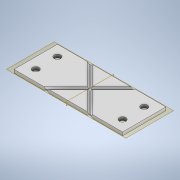
# Autodesk Inventor part: test_hangle_org_1
Saved by Autodesk Inventor 2020 (Build 240168000, 168)
## iProperties
Created: 2021-04-08
Part Number: test_hangle_org_1
Material: Generic
Document SubType Name: Modeling
Designer: Shuang Peng
Density: 1 g/cm^3
Appearance: Default
Author: Shuang Peng
Autodesk Inventor part; units mm, degrees
ref_plane "YZ Plane" through (0, 0, 0) normal (1, 0, 0) x (0, 1, 0)
ref_plane "XZ Plane" through (0, 0, 0) normal (0, 1, 0) x (-1, 0, 0)
ref_plane "XY Plane" through (0, 0, 0) normal (0, 0, 1) x (1, 0, 0)
sketch "Sketch1" plane through (0, 0, 0) normal (0, 1, 0) x (-1, 0, 0)
  line L0 (0, 0) -> (50, 0)
  line L1 (50, 0) -> (50, -20)
  line L2 (50, -20) -> (0, -20)
  line L3 (0, -20) -> (0, 0)
  line L4 (25, 0) -> (25, -20)
  line L5 (25, -20) -> (35, -20)
  line L6 (25, 0) -> (35, 0)
  line L7 (25, 0) -> (15, 0)
  line L8 (25, -20) -> (15, -20)
  line L9 (15, -20) -> (25, -10)
  line L10 (15, 0) -> (25, -10)
  line L11 (25, -10) -> (35, -20)
  line L12 (25, -10) -> (35, 0)
  line L13 (39.318912, 3.965359) -> (38.965359, 4.318912)
  line L14 (38.965359, 4.318912) -> (10.681088, -23.965359)
  line L15 (10.681088, -23.965359) -> (11.034641, -24.318912)
  line L16 (11.034641, -24.318912) -> (39.318912, 3.965359)
  line L17 (39.318912, 3.965359) -> (10.681088, -23.965359) construction
  line L18 (38.965359, 4.318912) -> (11.034641, -24.318912) construction
  line L19 (39.318912, -23.965359) -> (38.965359, -24.318912)
  line L20 (38.965359, -24.318912) -> (10.681088, 3.965359)
  line L21 (10.681088, 3.965359) -> (11.034641, 4.318912)
  line L22 (11.034641, 4.318912) -> (39.318912, -23.965359)
  line L23 (39.318912, -23.965359) -> (10.681088, 3.965359) construction
  line L24 (38.965359, -24.318912) -> (11.034641, 4.318912) construction
  point P0 (14.646447, -20)
  point P1 (24.646447, -10)
  point P2 (14.646447, 0)
  point P3 (35.353553, 0)
  point P4 (25.353553, -10)
  point P5 (35.353553, -20)
  point P6 (25, -10.353553)
  point P7 (15.353553, -20)
  point P8 (34.646447, -20)
  point P9 (15.353553, 0)
  point P10 (25, -9.646447)
  point P11 (34.646447, 0)
  dimension "d0" = 50
  dimension "d1" = 20
  dimension "d2" = 10
  dimension "d3" = 10
  dimension "d4" = 10
  dimension "d5" = 10
  dimension "d6" = 0.5
  dimension "d7" = 40
  dimension "d8" = 0.5
  dimension "d9" = 40
  constraints: 50 end point, 7 midpoint, 6 parallel, 5 perpendicular, 4 point on line, 1 horizontal
  measures "d0" distance of L1.end L2.end
  measures "d1" distance of L0.end L1.end
  measures "d2" distance of L4.end L5.end
  measures "d3" distance of L4.start L6.end
  measures "d4" distance of L4.start L7.end
  measures "d5" distance of L4.end L8.end
  measures "d6" distance of L13.start L13.end
  measures "d7" distance of L14.end L13.end
  measures "d8" distance of L19.start L19.end
  measures "d9" distance of L19.end L20.end
extrude "Extrusion1" add sketch "Sketch1" along normal blind 1.5 contours L0 L20 L14 L2 L3 | L0 L4 L22 | L0 L14 L4 | L20 L2 L4 | L4 L2 L16 | L16 L0 L1 L2 L22
ref_plane "Work Plane1" through (0, 0.75, 0) normal (0, 1, 0) x (1, 0, 0)
sketch "Sketch2" plane through (0, 0.75, 0) normal (0, 1, 0) x (1, 0, 0)
  line L0 (-14.646447, 0) -> (0, 0)
  line L1 (-24.646447, 10) -> (-14.646447, 0)
  line L2 (-14.646447, 20) -> (-24.646447, 10)
  line L3 (0, 20) -> (-14.646447, 20)
  line L4 (0, 0) -> (0, 20)
  line L5 (-15.353553, 20) -> (-34.646447, 20)
  line L6 (-25, 10.353553) -> (-15.353553, 20)
  line L7 (-34.646447, 20) -> (-25, 10.353553)
  line L8 (-35.353553, 0) -> (-25.353553, 10)
  line L9 (-50, 0) -> (-35.353553, 0)
  line L10 (-50, 20) -> (-50, 0)
  line L11 (-35.353553, 20) -> (-50, 20)
  line L12 (-25.353553, 10) -> (-35.353553, 20)
  line L13 (-34.646447, 0) -> (-15.353553, 0)
  line L14 (-25, 9.646447) -> (-34.646447, 0)
  line L15 (-15.353553, 0) -> (-25, 9.646447)
  line L16 (0, 0) -> (-50, 0)
  line L17 (0, 20) -> (-50, 20)
  constraints: 4 end point, 2 horizontal
extrude "Extrusion2" add sketch "Sketch2" along normal mid plane 0.15 contours L16 L15 L14 L8 L12 L17 L7 L6 L2 L1
chamfer "Chamfer1" distance 0.675 angle 45 16 edges at (-20.1768, 0, -15.1768) (-19.6464, 0, -15) (-29.8232, 0, -15.1768) (-30.3536, 0, -15) (-30.3536, 0, -5) (-29.8232, 0, -4.8232) (-20.1768, 0, -4.8232) (-19.6464, 0, -5) (-19.6464, 1.5, -15) (-20.1768, 1.5, -15.1768) (-29.8232, 1.5, -15.1768) (-30.3536, 1.5, -15) (-30.3536, 1.5, -5) (-29.8232, 1.5, -4.8232) (-20.1768, 1.5, -4.8232) (-19.6464, 1.5, -5)
sketch "Sketch3" plane through (0, 0, 0) normal (0, -1, 0) x (1, 0, 0)
  line L0 (-23.691852, -10) -> (-13.691852, 0)
  line L1 (-13.691852, -20) -> (-23.691852, -10)
  line L2 (0, -20) -> (-13.691852, -20)
  line L3 (0, 0) -> (0, -20)
  line L4 (-13.691852, 0) -> (0, 0)
  line L5 (-36.308148, 0) -> (-26.308148, -10)
  line L6 (-50, 0) -> (-36.308148, 0)
  line L7 (-50, -20) -> (-50, 0)
  line L8 (-36.308148, -20) -> (-50, -20)
  line L9 (-26.308148, -10) -> (-36.308148, -20)
  line L10 (0, 0) -> (0, -20)
  line L11 (0, -10) -> (-5, -10)
  line L12 (-5, -10) -> (-5, -15)
  line L13 (-5, -10) -> (-5, -5)
  circle A0 centre (-5, -15) radius 1.5
  circle A1 centre (-5, -5) radius 1.5
  dimension "d17" = 5
  dimension "d18" = 5
  dimension "d19" = 5
  dimension "d20" = 3
  dimension "d21" = 3
  constraints: 6 end point, 2 centre point, 2 coincident, 1 horizontal, 1 midpoint, 1 perpendicular, 1 vertical
  measures "d17" distance of L11.start L11.end
  measures "d18" distance of L11.end L12.end
  measures "d19" distance of L11.end L13.end
  measures "d20" diameter of A0
  measures "d21" diameter of A1
extrude "Extrusion3" cut sketch "Sketch3" against normal blind 4 contours A0 | A1
ref_plane "Work Plane2" through (-25, 0, 0) normal (1, 0, 0) x (0, 0, -1)
mirror "Mirror1" about plane through (-25, 0, 0) normal (1, 0, 0) of "Extrusion3"
thicken "Thicken1" operation add thickness 0.07 both sides no extend neighbours yes toward (0, 1, 0) faces at (-18.215482, 0.825, -16.666667)
thicken "Thicken2" operation add thickness 0.07 both sides no extend neighbours yes toward (0, -1, 0) faces at (-18.215482, 0.675, -16.666667)
body "Solid1"
